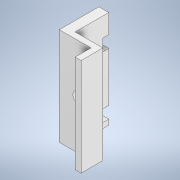
# Autodesk Inventor part: Base Idler Izq
Saved by Autodesk Inventor 2021 (Build 250183000, 183)
## iProperties
Created: 2023-01-27
Part Number: Base Idler Izq
Material: Plástico PAEK
Document SubType Name: Modeling
Designer: Diego.labarca
Density: 1.32 g/cm^3
Appearance: Suave - Blanco
Author: Diego.labarca
Autodesk Inventor part; units mm, degrees
ref_plane "YZ Plane" through (0, 0, 0) normal (1, 0, 0) x (0, 1, 0)
ref_plane "XZ Plane" through (0, 0, 0) normal (0, 1, 0) x (-1, 0, 0)
ref_plane "XY Plane" through (0, 0, 0) normal (0, 0, 1) x (1, 0, 0)
sketch "Boceto15" plane through (0, 0, 0) normal (1, 0, 0) x (0, 1, 0)
  line L0 (24.65, 10) -> (-24.65, 10)
  line L1 (-24.65, 10) -> (-24.65, -10)
  line L2 (-24.65, -10) -> (24.65, -10)
  line L3 (24.65, -10) -> (24.65, 10)
  line L4 (0, -2.1261) -> (0, 0)
  line L5 (0, 0) -> (1.5481, 0)
  dimension "d52" = 49.3
  dimension "d53" = 20
  constraints: 12 end point, 2 parallel, 2 perpendicular, 1 horizontal, 1 vertical, 2 other
  measures "d52" distance of L2.end L1.end
  measures "d53" distance of L1.end L0.end
extrude "Extrusión12" add sketch "Boceto15" along normal blind 5
sketch "Boceto16" plane through (5, 0, 0) normal (1, 0, 0) x (0, 0, -1)
  circle A0 centre (3.5, -14.65) radius 1.5
  line L0 (10, -24.65) -> (10, 24.65) projected
  line L1 (-10, -24.65) -> (10, -24.65) projected
  circle A1 centre (3.5, 7.35) radius 1.5
  point P0 (0, 0)
  dimension "d56" = 6.5
  dimension "d57" = 10
  dimension "d58" = 3
  dimension "d59" = 3
  dimension "d60" = 32
  dimension "d61" = 6.5
  constraints: 2 centre point
  measures "d56" distance from line of A0.centre L0
  measures "d57" distance from line of L1 A0.centre
  measures "d58" diameter of A0
  measures "d59" diameter of A1
  measures "d60" distance from line of L1 A1.centre
  measures "d61" distance from line of A1.centre L0
extrude "Extrusión13" cut sketch "Boceto16" against normal through all
sketch "Boceto17" plane through (0, -24.65, -10) normal (0, -1, 0) x (1, 0, 0)
  line L0 (5, 20) -> (5, 0) projected
  line L1 (5, 20) -> (16, 20)
  line L2 (16, 20) -> (16, 17)
  line L3 (16, 17) -> (5, 17)
  line L4 (5, 17) -> (5, 20)
  line L5 (16, 17) -> (19, 17)
  line L6 (19, 17) -> (19, 28)
  line L7 (19, 28) -> (16, 28)
  line L8 (16, 28) -> (16, 17)
  point P0 (0, 10)
  dimension "d64" = 11
  dimension "d65" = 3
  dimension "d66" = 3
  dimension "d67" = 11
  constraints: 16 end point, 4 parallel, 2 horizontal, 2 perpendicular
  measures "d64" distance of L2.end L3.end
  measures "d65" distance of L1.end L2.end
  measures "d66" distance of L7.end L6.end
  measures "d67" distance of L6.end L5.end
extrude "Extrusión14" add sketch "Boceto17" against normal up to surface (49.3 mm away)
sketch "Boceto18" plane through (0, -24.65, 10) normal (0, 0, 1) x (1, 0, 0)
  circle A0 centre (10, 24.3) radius 3.134
  line L0 (0, 0) -> (16, 0) projected
  line L1 (0, 49.3) -> (0, 0) projected
  point P0 (0, 24.65)
  dimension "d70" = 24.3
  dimension "d71" = 10
  constraints: 1 centre point
  measures "d70" distance from line of A0.centre L0
  measures "d71" distance from line of L1 A0.centre
extrude "Extrusión15" cut sketch "Boceto18" against normal up to surface (3 mm away)
sketch "Boceto19" plane through (5, 0, 0) normal (1, 0, 0) x (0, 0, -1)
  line L0 (10, -24.65) -> (10, 24.65) projected
  line L1 (10, -22) -> (7, -22)
  line L2 (7, -22) -> (7, -16)
  line L3 (7, -16) -> (10, -16)
  line L4 (10, -16) -> (10, -22)
  line L5 (10, 9) -> (7, 9)
  line L6 (7, 9) -> (7, 15)
  line L7 (7, 15) -> (10, 15)
  line L8 (10, 15) -> (10, 9)
  line L9 (7, 12) -> (8.4797, 12)
  line L10 (7, -19) -> (9.1788, -19)
  line L11 (-7, -24.65) -> (10, -24.65) projected
  point P0 (0, 0)
  dimension "d74" = 5.65
  dimension "d75" = 6
  dimension "d76" = 6
  dimension "d77" = 31
  dimension "d78" = 3
  constraints: 20 end point, 4 horizontal, 4 parallel, 3 point on line, 2 midpoint, 2 perpendicular
  measures "d74" distance between parallel lines of L11 L10
  measures "d75" distance of L1.end L2.end
  measures "d76" distance of L5.end L6.end
  measures "d77" distance between parallel lines of L10 L9
  measures "d78" distance of L2.end L3.end
extrude "Extrusión16" cut sketch "Boceto19" against normal through all
equation "\"d59\" = d58"
equation "\"d61\" = d56"
equation "\"d68\" = d65"
equation "\"d76\" = d75"
